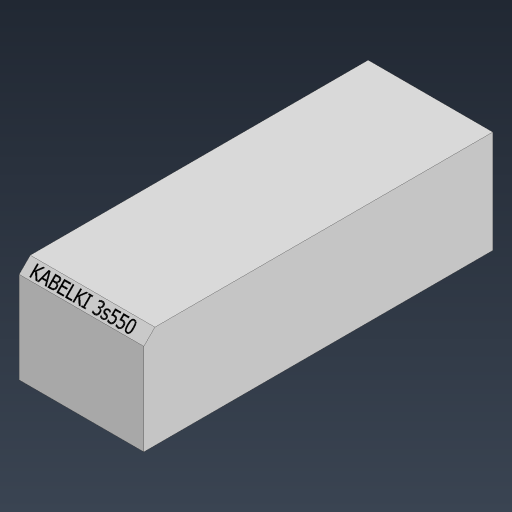
# Autodesk Inventor part: 2s450mah
Saved by Autodesk Inventor 2023 (Build 270158000, 158)
## iProperties
Created: 2026-03-09
Part Number: 2s450mah
Material: Generic
Document SubType Name: Modeling
Designer: szymo
Density: 1 g/cm^3
Appearance: Default
Author: szymo
Autodesk Inventor part; units mm, degrees
ref_plane "YZ Plane" through (0, 0, 0) normal (1, 0, 0) x (0, 1, 0)
ref_plane "XZ Plane" through (0, 0, 0) normal (0, 1, 0) x (-1, 0, 0)
ref_plane "XY Plane" through (0, 0, 0) normal (0, 0, 1) x (1, 0, 0)
sketch "Sketch1" plane through (0, 0, 0) normal (0, 1, 0) x (-1, 0, 0)
  line L0 (0, 0) -> (-22.5, 0)
  line L1 (-22.5, 0) -> (-22.5, -63)
  line L2 (-22.5, -63) -> (0, -63)
  line L3 (0, -63) -> (0, 0)
  dimension "d0" = 22.5
  dimension "d1" = 63
  constraints: 8 end point, 2 parallel, 1 horizontal, 1 perpendicular
  measures "d0" distance of L2.end L1.end
  measures "d1" distance of L0.end L1.end
extrude "Extrusion1" add sketch "Sketch1" along normal blind 18.5
chamfer "Chamfer1" distance 2 angle 45 1 edges at (11.25, 18.5, 0)
sketch "Sketch2" plane through (0, 18.5, -2) normal (0, 0.7071, 0.7071) x (1, 0, 0)
  line L0 (1.3725, -0.4182) -> (25.1586, -0.4182) construction
  line L1 (25.1586, -0.4182) -> (25.1586, -2.7468) construction
  line L2 (25.1586, -2.7468) -> (1.3725, -2.7468) construction
  line L3 (1.3725, -2.7468) -> (1.3725, -0.4182) construction
  line L4 (3.0338, -2.4603) -> (2.6886, -2.4603)
  line L5 (2.6886, -2.4603) -> (1.9576, -1.53)
  line L6 (1.9576, -1.53) -> (1.8409, -1.6613)
  line L7 (1.8409, -1.6613) -> (1.8409, -2.4603)
  line L8 (1.8409, -2.4603) -> (1.5751, -2.4603)
  line L9 (1.5751, -2.4603) -> (1.5751, -0.4603)
  line L10 (1.5751, -0.4603) -> (1.8409, -0.4603)
  line L11 (1.8409, -0.4603) -> (1.8409, -1.3793)
  line L12 (1.8409, -1.3793) -> (2.661, -0.4603)
  line L13 (2.661, -0.4603) -> (2.9851, -0.4603)
  line L14 (2.9851, -0.4603) -> (2.1569, -1.3534)
  line L15 (2.1569, -1.3534) -> (3.0338, -2.4603)
  line L16 (2.977, -2.4603) -> (3.6513, -0.4603)
  line L17 (3.6513, -0.4603) -> (3.9787, -0.4603)
  line L18 (3.9787, -0.4603) -> (4.6529, -2.4603)
  line L19 (4.6529, -2.4603) -> (4.3725, -2.4603)
  line L20 (4.3725, -2.4603) -> (4.191, -1.9012)
  line L21 (4.191, -1.9012) -> (3.4276, -1.9012)
  line L22 (3.4276, -1.9012) -> (3.2461, -2.4603)
  line L23 (3.2461, -2.4603) -> (2.977, -2.4603)
  line L24 (4.118, -1.6743) -> (3.8085, -0.7326)
  line L25 (3.8085, -0.7326) -> (3.5005, -1.6743)
  line L26 (3.5005, -1.6743) -> (4.118, -1.6743)
  spline S0 degree 2 poles (6.1991, -1.8461) (6.1991, -1.9952) (6.0856, -2.2237) (5.9916, -2.2983) knots 0 0 0 1 2 2 2
  spline S1 degree 2 poles (5.9916, -2.2983) (5.8782, -2.3858) (5.6205, -2.4603) (5.4163, -2.4603) knots 0 0 0 1 2 2 2
  line L27 (5.4163, -2.4603) -> (4.8425, -2.4603)
  line L28 (4.8425, -2.4603) -> (4.8425, -0.4603)
  line L29 (4.8425, -0.4603) -> (5.3725, -0.4603)
  spline S2 degree 2 poles (5.3725, -0.4603) (5.5864, -0.4603) (5.8004, -0.4879) (5.8976, -0.5414) knots 0 0 0 1 2 2 2
  spline S3 degree 2 poles (5.8976, -0.5414) (6.0062, -0.5981) (6.1051, -0.7845) (6.1051, -0.9109) knots 0 0 0 1 2 2 2
  spline S4 degree 2 poles (6.1051, -0.9109) (6.1051, -1.0519) (5.956, -1.2756) (5.8247, -1.3388) knots 0 0 0 1 2 2 2
  line L30 (5.8247, -1.3388) -> (5.8247, -1.3485)
  spline S5 degree 2 poles (5.8247, -1.3485) (6.003, -1.3971) (6.1991, -1.6548) (6.1991, -1.8461) knots 0 0 0 1 2 2 2
  spline S6 degree 2 poles (5.9219, -1.8574) (5.9219, -1.744) (5.8571, -1.5981) (5.7599, -1.5462) knots 0 0 0 1 2 2 2
  spline S7 degree 2 poles (5.7599, -1.5462) (5.6967, -1.5138) (5.5475, -1.4944) (5.4098, -1.4944) knots 0 0 0 1 2 2 2
  line L31 (5.4098, -1.4944) -> (5.1083, -1.4944)
  line L32 (5.1083, -1.4944) -> (5.1083, -2.2334)
  line L33 (5.1083, -2.2334) -> (5.3239, -2.2334)
  spline S8 degree 2 poles (5.3239, -2.2334) (5.4989, -2.2334) (5.6999, -2.201) (5.7777, -2.1491) knots 0 0 0 1 2 2 2
  spline S9 degree 2 poles (5.7777, -2.1491) (5.8522, -2.0957) (5.9219, -1.9628) (5.9219, -1.8574) knots 0 0 0 1 2 2 2
  spline S10 degree 2 poles (5.8279, -0.9482) (5.8279, -0.8769) (5.7793, -0.7699) (5.7258, -0.7391) knots 0 0 0 1 2 2 2
  spline S11 degree 2 poles (5.7258, -0.7391) (5.661, -0.7034) (5.5038, -0.6872) (5.3628, -0.6872) knots 0 0 0 1 2 2 2
  line L34 (5.3628, -0.6872) -> (5.1083, -0.6872)
  line L35 (5.1083, -0.6872) -> (5.1083, -1.2723)
  line L36 (5.1083, -1.2723) -> (5.4098, -1.2723)
  spline S12 degree 2 poles (5.4098, -1.2723) (5.5346, -1.2723) (5.6529, -1.2464) (5.7161, -1.2059) knots 0 0 0 1 2 2 2
  spline S13 degree 2 poles (5.7161, -1.2059) (5.7777, -1.167) (5.8279, -1.0422) (5.8279, -0.9482) knots 0 0 0 1 2 2 2
  line L37 (6.4633, -2.4603) -> (6.4633, -0.4603)
  line L38 (6.4633, -0.4603) -> (7.7145, -0.4603)
  line L39 (7.7145, -0.4603) -> (7.7145, -0.697)
  line L40 (7.7145, -0.697) -> (6.7291, -0.697)
  line L41 (6.7291, -0.697) -> (6.7291, -1.2448)
  line L42 (6.7291, -1.2448) -> (7.648, -1.2448)
  line L43 (7.648, -1.2448) -> (7.648, -1.4814)
  line L44 (7.648, -1.4814) -> (6.7291, -1.4814)
  line L45 (6.7291, -1.4814) -> (6.7291, -2.2237)
  line L46 (6.7291, -2.2237) -> (7.7145, -2.2237)
  line L47 (7.7145, -2.2237) -> (7.7145, -2.4603)
  line L48 (7.7145, -2.4603) -> (6.4633, -2.4603)
  line L49 (9.1651, -2.4603) -> (8.0062, -2.4603)
  line L50 (8.0062, -2.4603) -> (8.0062, -0.4603)
  line L51 (8.0062, -0.4603) -> (8.272, -0.4603)
  line L52 (8.272, -0.4603) -> (8.272, -2.2237)
  line L53 (8.272, -2.2237) -> (9.1651, -2.2237)
  line L54 (9.1651, -2.2237) -> (9.1651, -2.4603)
  line L55 (10.8328, -2.4603) -> (10.4876, -2.4603)
  line L56 (10.4876, -2.4603) -> (9.7566, -1.53)
  line L57 (9.7566, -1.53) -> (9.6399, -1.6613)
  line L58 (9.6399, -1.6613) -> (9.6399, -2.4603)
  line L59 (9.6399, -2.4603) -> (9.3741, -2.4603)
  line L60 (9.3741, -2.4603) -> (9.3741, -0.4603)
  line L61 (9.3741, -0.4603) -> (9.6399, -0.4603)
  line L62 (9.6399, -0.4603) -> (9.6399, -1.3793)
  line L63 (9.6399, -1.3793) -> (10.46, -0.4603)
  line L64 (10.46, -0.4603) -> (10.7842, -0.4603)
  line L65 (10.7842, -0.4603) -> (9.956, -1.3534)
  line L66 (9.956, -1.3534) -> (10.8328, -2.4603)
  line L67 (11.6886, -2.4603) -> (10.9138, -2.4603)
  line L68 (10.9138, -2.4603) -> (10.9138, -2.2561)
  line L69 (10.9138, -2.2561) -> (11.1683, -2.2561)
  line L70 (11.1683, -2.2561) -> (11.1683, -0.6645)
  line L71 (11.1683, -0.6645) -> (10.9138, -0.6645)
  line L72 (10.9138, -0.6645) -> (10.9138, -0.4603)
  line L73 (10.9138, -0.4603) -> (11.6886, -0.4603)
  line L74 (11.6886, -0.4603) -> (11.6886, -0.6645)
  line L75 (11.6886, -0.6645) -> (11.4341, -0.6645)
  line L76 (11.4341, -0.6645) -> (11.4341, -2.2561)
  line L77 (11.4341, -2.2561) -> (11.6886, -2.2561)
  line L78 (11.6886, -2.2561) -> (11.6886, -2.4603)
  spline S14 degree 2 poles (13.3595, -0.65) (13.2866, -0.65) (13.1424, -0.6856) (13.0727, -0.7132) knots 0 0 0 1 2 2 2
  spline S15 degree 2 poles (13.0727, -0.7132) (13.0078, -0.7407) (12.9122, -0.7991) (12.8749, -0.825) knots 0 0 0 1 2 2 2
  line L79 (12.8749, -0.825) -> (12.8587, -0.825)
  line L80 (12.8587, -0.825) -> (12.8587, -0.5414)
  spline S16 degree 2 poles (12.8587, -0.5414) (12.9463, -0.4944) (13.2461, -0.4182) (13.3806, -0.4182) knots 0 0 0 1 2 2 2
  spline S17 degree 2 poles (13.3806, -0.4182) (13.5168, -0.4182) (13.7193, -0.4733) (13.802, -0.5316) knots 0 0 0 1 2 2 2
  spline S18 degree 2 poles (13.802, -0.5316) (13.8895, -0.5948) (13.9803, -0.778) (13.9803, -0.9012) knots 0 0 0 1 2 2 2
  spline S19 degree 2 poles (13.9803, -0.9012) (13.9803, -1.0665) (13.7631, -1.3161) (13.6108, -1.3485) knots 0 0 0 1 2 2 2
  line L81 (13.6108, -1.3485) -> (13.6108, -1.3679)
  spline S20 degree 2 poles (13.6108, -1.3679) (13.674, -1.3809) (13.8182, -1.4393) (13.8798, -1.4976) knots 0 0 0 1 2 2 2
  spline S21 degree 2 poles (13.8798, -1.4976) (13.9414, -1.5543) (14.0192, -1.7359) (14.0192, -1.8671) knots 0 0 0 1 2 2 2
  spline S22 degree 2 poles (14.0192, -1.8671) (14.0192, -2.0017) (13.9268, -2.2302) (13.8425, -2.3177) knots 0 0 0 1 2 2 2
  spline S23 degree 2 poles (13.8425, -2.3177) (13.755, -2.4085) (13.507, -2.5025) (13.3498, -2.5025) knots 0 0 0 1 2 2 2
  spline S24 degree 2 poles (13.3498, -2.5025) (13.1991, -2.5025) (12.9041, -2.4295) (12.8036, -2.3793) knots 0 0 0 1 2 2 2
  line L82 (12.8036, -2.3793) -> (12.8036, -2.0957)
  line L83 (12.8036, -2.0957) -> (12.8231, -2.0957)
  spline S25 degree 2 poles (12.8231, -2.0957) (12.9074, -2.1572) (13.1926, -2.2707) (13.3336, -2.2707) knots 0 0 0 1 2 2 2
  spline S26 degree 2 poles (13.3336, -2.2707) (13.4163, -2.2707) (13.5816, -2.2188) (13.6367, -2.1589) knots 0 0 0 1 2 2 2
  spline S27 degree 2 poles (13.6367, -2.1589) (13.6902, -2.0989) (13.7469, -1.9563) (13.7469, -1.8477) knots 0 0 0 1 2 2 2
  spline S28 degree 2 poles (13.7469, -1.8477) (13.7469, -1.7391) (13.6837, -1.5981) (13.627, -1.5576) knots 0 0 0 1 2 2 2
  spline S29 degree 2 poles (13.627, -1.5576) (13.5702, -1.5171) (13.4163, -1.4863) (13.3255, -1.4863) knots 0 0 0 1 2 2 2
  line L84 (13.3255, -1.4863) -> (13.2121, -1.4863)
  line L85 (13.2121, -1.4863) -> (13.2121, -1.2642)
  line L86 (13.2121, -1.2642) -> (13.3012, -1.2642)
  spline S30 degree 2 poles (13.3012, -1.2642) (13.4811, -1.2642) (13.708, -1.0924) (13.708, -0.9287) knots 0 0 0 1 2 2 2
  spline S31 degree 2 poles (13.708, -0.9287) (13.708, -0.8525) (13.6497, -0.744) (13.6027, -0.7115) knots 0 0 0 1 2 2 2
  spline S32 degree 2 poles (13.6027, -0.7115) (13.5524, -0.6775) (13.4292, -0.65) (13.3595, -0.65) knots 0 0 0 1 2 2 2
  spline S33 degree 2 poles (14.7631, -2.496) (14.6124, -2.496) (14.3514, -2.4149) (14.2655, -2.3696) knots 0 0 0 1 2 2 2
  line L87 (14.2655, -2.3696) -> (14.2655, -2.0859)
  line L88 (14.2655, -2.0859) -> (14.2785, -2.0859)
  spline S34 degree 2 poles (14.2785, -2.0859) (14.3109, -2.1119) (14.3984, -2.1735) (14.4714, -2.2075) knots 0 0 0 1 2 2 2
  spline S35 degree 2 poles (14.4714, -2.2075) (14.5346, -2.2383) (14.6902, -2.2837) (14.7728, -2.2837) knots 0 0 0 1 2 2 2
  spline S36 degree 2 poles (14.7728, -2.2837) (14.8328, -2.2837) (14.9706, -2.2561) (15.003, -2.2334) knots 0 0 0 1 2 2 2
  spline S37 degree 2 poles (15.003, -2.2334) (15.05, -2.2026) (15.0921, -2.1329) (15.0921, -2.0616) knots 0 0 0 1 2 2 2
  spline S38 degree 2 poles (15.0921, -2.0616) (15.0921, -1.9725) (14.9949, -1.8801) (14.8701, -1.8493) knots 0 0 0 1 2 2 2
  spline S39 degree 2 poles (14.8701, -1.8493) (14.8215, -1.838) (14.6659, -1.8055) (14.5994, -1.7877) knots 0 0 0 1 2 2 2
  spline S40 degree 2 poles (14.5994, -1.7877) (14.4276, -1.7375) (14.272, -1.53) (14.272, -1.3825) knots 0 0 0 1 2 2 2
  spline S41 degree 2 poles (14.272, -1.3825) (14.272, -1.1783) (14.5783, -0.9239) (14.8312, -0.9239) knots 0 0 0 1 2 2 2
  spline S42 degree 2 poles (14.8312, -0.9239) (14.956, -0.9239) (15.2088, -0.9854) (15.2947, -1.0325) knots 0 0 0 1 2 2 2
  line L89 (15.2947, -1.0325) -> (15.2947, -1.3031)
  line L90 (15.2947, -1.3031) -> (15.2817, -1.3031)
  spline S43 degree 2 poles (15.2817, -1.3031) (15.1845, -1.2253) (14.9479, -1.1362) (14.8263, -1.1362) knots 0 0 0 1 2 2 2
  spline S44 degree 2 poles (14.8263, -1.1362) (14.7015, -1.1362) (14.5297, -1.2415) (14.5297, -1.3469) knots 0 0 0 1 2 2 2
  spline S45 degree 2 poles (14.5297, -1.3469) (14.5297, -1.4425) (14.6318, -1.5349) (14.7453, -1.5641) knots 0 0 0 1 2 2 2
  spline S46 degree 2 poles (14.7453, -1.5641) (14.8004, -1.5786) (14.9398, -1.6078) (15.0159, -1.6256) knots 0 0 0 1 2 2 2
  spline S47 degree 2 poles (15.0159, -1.6256) (15.1813, -1.6678) (15.3498, -1.8607) (15.3498, -2.0276) knots 0 0 0 1 2 2 2
  spline S48 degree 2 poles (15.3498, -2.0276) (15.3498, -2.1248) (15.2736, -2.2966) (15.1991, -2.3598) knots 0 0 0 1 2 2 2
  spline S49 degree 2 poles (15.1991, -2.3598) (15.1197, -2.4263) (14.9171, -2.496) (14.7631, -2.496) knots 0 0 0 1 2 2 2
  spline S50 degree 2 poles (16.7599, -1.825) (16.7599, -1.9692) (16.6675, -2.2156) (16.5832, -2.3064) knots 0 0 0 1 2 2 2
  spline S51 degree 2 poles (16.5832, -2.3064) (16.4989, -2.3971) (16.2477, -2.5025) (16.0921, -2.5025) knots 0 0 0 1 2 2 2
  spline S52 degree 2 poles (16.0921, -2.5025) (15.9495, -2.5025) (15.6707, -2.4393) (15.5686, -2.389) knots 0 0 0 1 2 2 2
  line L91 (15.5686, -2.389) -> (15.5686, -2.1054)
  line L92 (15.5686, -2.1054) -> (15.5881, -2.1054)
  spline S53 degree 2 poles (15.5881, -2.1054) (15.6189, -2.1281) (15.7339, -2.1864) (15.8036, -2.2124) knots 0 0 0 1 2 2 2
  spline S54 degree 2 poles (15.8036, -2.2124) (15.883, -2.2399) (16.0143, -2.2707) (16.097, -2.2707) knots 0 0 0 1 2 2 2
  spline S55 degree 2 poles (16.097, -2.2707) (16.178, -2.2707) (16.3304, -2.2124) (16.3855, -2.1491) knots 0 0 0 1 2 2 2
  spline S56 degree 2 poles (16.3855, -2.1491) (16.4357, -2.0892) (16.4876, -1.9303) (16.4876, -1.8234) knots 0 0 0 1 2 2 2
  spline S57 degree 2 poles (16.4876, -1.8234) (16.4876, -1.7164) (16.4292, -1.5803) (16.3741, -1.5349) knots 0 0 0 1 2 2 2
  spline S58 degree 2 poles (16.3741, -1.5349) (16.3174, -1.4846) (16.1488, -1.4425) (16.0467, -1.4425) knots 0 0 0 1 2 2 2
  spline S59 degree 2 poles (16.0467, -1.4425) (15.9365, -1.4425) (15.7177, -1.4765) (15.6513, -1.4911) knots 0 0 0 1 2 2 2
  line L93 (15.6513, -1.4911) -> (15.6513, -0.4603)
  line L94 (15.6513, -0.4603) -> (16.7485, -0.4603)
  line L95 (16.7485, -0.4603) -> (16.7485, -0.6953)
  line L96 (16.7485, -0.6953) -> (15.909, -0.6953)
  line L97 (15.909, -0.6953) -> (15.909, -1.2286)
  spline S60 degree 2 poles (15.909, -1.2286) (15.9576, -1.2221) (16.0516, -1.2172) (16.0905, -1.2172) knots 0 0 0 1 2 2 2
  spline S61 degree 2 poles (16.0905, -1.2172) (16.2445, -1.2172) (16.4568, -1.2675) (16.554, -1.342) knots 0 0 0 1 2 2 2
  spline S62 degree 2 poles (16.554, -1.342) (16.6529, -1.4166) (16.7599, -1.6435) (16.7599, -1.825) knots 0 0 0 1 2 2 2
  spline S63 degree 2 poles (18.2607, -1.825) (18.2607, -1.9692) (18.1683, -2.2156) (18.084, -2.3064) knots 0 0 0 1 2 2 2
  spline S64 degree 2 poles (18.084, -2.3064) (17.9997, -2.3971) (17.7485, -2.5025) (17.5929, -2.5025) knots 0 0 0 1 2 2 2
  spline S65 degree 2 poles (17.5929, -2.5025) (17.4503, -2.5025) (17.1715, -2.4393) (17.0694, -2.389) knots 0 0 0 1 2 2 2
  line L98 (17.0694, -2.389) -> (17.0694, -2.1054)
  line L99 (17.0694, -2.1054) -> (17.0889, -2.1054)
  spline S66 degree 2 poles (17.0889, -2.1054) (17.1197, -2.1281) (17.2347, -2.1864) (17.3044, -2.2124) knots 0 0 0 1 2 2 2
  spline S67 degree 2 poles (17.3044, -2.2124) (17.3839, -2.2399) (17.5151, -2.2707) (17.5978, -2.2707) knots 0 0 0 1 2 2 2
  spline S68 degree 2 poles (17.5978, -2.2707) (17.6788, -2.2707) (17.8312, -2.2124) (17.8863, -2.1491) knots 0 0 0 1 2 2 2
  spline S69 degree 2 poles (17.8863, -2.1491) (17.9365, -2.0892) (17.9884, -1.9303) (17.9884, -1.8234) knots 0 0 0 1 2 2 2
  spline S70 degree 2 poles (17.9884, -1.8234) (17.9884, -1.7164) (17.93, -1.5803) (17.8749, -1.5349) knots 0 0 0 1 2 2 2
  spline S71 degree 2 poles (17.8749, -1.5349) (17.8182, -1.4846) (17.6497, -1.4425) (17.5475, -1.4425) knots 0 0 0 1 2 2 2
  spline S72 degree 2 poles (17.5475, -1.4425) (17.4373, -1.4425) (17.2185, -1.4765) (17.1521, -1.4911) knots 0 0 0 1 2 2 2
  line L100 (17.1521, -1.4911) -> (17.1521, -0.4603)
  line L101 (17.1521, -0.4603) -> (18.2493, -0.4603)
  line L102 (18.2493, -0.4603) -> (18.2493, -0.6953)
  line L103 (18.2493, -0.6953) -> (17.4098, -0.6953)
  line L104 (17.4098, -0.6953) -> (17.4098, -1.2286)
  spline S73 degree 2 poles (17.4098, -1.2286) (17.4584, -1.2221) (17.5524, -1.2172) (17.5913, -1.2172) knots 0 0 0 1 2 2 2
  spline S74 degree 2 poles (17.5913, -1.2172) (17.7453, -1.2172) (17.9576, -1.2675) (18.0548, -1.342) knots 0 0 0 1 2 2 2
  spline S75 degree 2 poles (18.0548, -1.342) (18.1537, -1.4166) (18.2607, -1.6435) (18.2607, -1.825) knots 0 0 0 1 2 2 2
  spline S76 degree 2 poles (19.7939, -1.4603) (19.7939, -1.9984) (19.4811, -2.5025) (19.1553, -2.5025) knots 0 0 0 1 2 2 2
  spline S77 degree 2 poles (19.1553, -2.5025) (18.8247, -2.5025) (18.5151, -1.9887) (18.5151, -1.4619) knots 0 0 0 1 2 2 2
  spline S78 degree 2 poles (18.5151, -1.4619) (18.5151, -0.9206) (18.8279, -0.4198) (19.1553, -0.4198) knots 0 0 0 1 2 2 2
  spline S79 degree 2 poles (19.1553, -0.4198) (19.4843, -0.4198) (19.7939, -0.9384) (19.7939, -1.4603) knots 0 0 0 1 2 2 2
  spline S80 degree 2 poles (19.4503, -2.0697) (19.4892, -1.9709) (19.5216, -1.6662) (19.5216, -1.4603) knots 0 0 0 1 2 2 2
  spline S81 degree 2 poles (19.5216, -1.4603) (19.5216, -1.2545) (19.4892, -0.9514) (19.4487, -0.8493) knots 0 0 0 1 2 2 2
  spline S82 degree 2 poles (19.4487, -0.8493) (19.4082, -0.7472) (19.2672, -0.6419) (19.1553, -0.6419) knots 0 0 0 1 2 2 2
  spline S83 degree 2 poles (19.1553, -0.6419) (19.0435, -0.6419) (18.8992, -0.7472) (18.8571, -0.8525) knots 0 0 0 1 2 2 2
  spline S84 degree 2 poles (18.8571, -0.8525) (18.8166, -0.9547) (18.7874, -1.2658) (18.7874, -1.4619) knots 0 0 0 1 2 2 2
  spline S85 degree 2 poles (18.7874, -1.4619) (18.7874, -1.6726) (18.8133, -1.9547) (18.8555, -2.0649) knots 0 0 0 1 2 2 2
  spline S86 degree 2 poles (18.8555, -2.0649) (18.8944, -2.1686) (19.0386, -2.2804) (19.1553, -2.2804) knots 0 0 0 1 2 2 2
  spline S87 degree 2 poles (19.1553, -2.2804) (19.2655, -2.2804) (19.4098, -2.1751) (19.4503, -2.0697) knots 0 0 0 1 2 2 2
  point P0 (0, -14.4957)
  constraints: 2 other
extrude "Extrusion2" cut sketch "Sketch2" against normal blind 1
body "Solid1"
